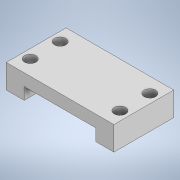
# Autodesk Inventor part: Controller_Strap
Saved by Autodesk Inventor 2022.3 (Build 263350000, 350)
## iProperties
Created: 2023-06-22
Part Number: Controller_Strap
Material: Generic
Document SubType Name: Modeling
Designer: natalie.jimenez
Density: 1 g/cm^3
Appearance: Default
Author: natalie.jimenez
Autodesk Inventor part; units mm, degrees
ref_plane "YZ Plane" through (0, 0, 0) normal (1, 0, 0) x (0, 1, 0)
ref_plane "XZ Plane" through (0, 0, 0) normal (0, 1, 0) x (-1, 0, 0)
ref_plane "XY Plane" through (0, 0, 0) normal (0, 0, 1) x (1, 0, 0)
sketch "Sketch1" plane through (0, 0, 0) normal (0, 1, 0) x (-1, 0, 0)
  line L0 (-11.43, -6.35) -> (11.43, -6.35)
  line L1 (11.43, -6.35) -> (11.43, 6.35)
  line L2 (11.43, 6.35) -> (-11.43, 6.35)
  line L3 (-11.43, 6.35) -> (-11.43, -6.35)
  line L4 (-11.43, -6.35) -> (11.43, 6.35) construction
  line L5 (11.43, -6.35) -> (-11.43, 6.35) construction
  point P0 (0, 0)
  point P1 (0, 0)
  dimension "d19" = 22.86
  dimension "d20" = 12.7
  constraints: 12 end point, 2 parallel, 1 coincident, 1 horizontal, 1 midpoint, 1 perpendicular
  measures "d19" distance between parallel lines of L3 L1
  measures "d20" distance between parallel lines of L0 L2
sketch "Sketch2" plane through (0, 0, 0) normal (0, 1, 0) x (-1, 0, 0)
  line L0 (9.525, 3.1634) -> (9.525, -3.1866) construction
  line L1 (9.525, -3.1866) -> (-9.525, -3.1866) construction
  line L2 (-9.525, -3.1866) -> (-9.525, 3.1634) construction
  line L3 (-9.525, 3.1634) -> (9.525, 3.1634) construction
  line L4 (9.525, 6.3268) -> (9.525, 3.1634) construction
  line L5 (-9.525, 3.1634) -> (-9.525, 6.5546) construction
  line L6 (11.43, -6.35) -> (11.43, 6.35) projected
  line L7 (-11.43, -6.35) -> (11.43, -6.35) projected
  line L8 (-11.43, 6.35) -> (-11.43, -6.35) projected
  line L9 (11.43, 6.35) -> (-11.43, 6.35) projected
  line L10 (9.525, -3.1866) -> (9.525, -6.35) construction
  point P0 (0, 0)
  dimension "d18" = 6.35
  dimension "d22" = 19.05
  dimension "d23" = 1.905
  dimension "d24" = 3.1634
  constraints: 14 end point, 4 perpendicular, 3 point on line, 2 collinear, 1 vertical
  measures "d18" distance between parallel lines of L1 L3
  measures "d22" distance between parallel lines of L2 L0
  measures "d23" distance between parallel lines of L6 L0
  measures "d24" distance between parallel lines of L1 L7
extrude "Extrusion1" add sketch "Sketch1" along normal blind 5.08
hole "Hole1" at (-9.525, 0, 3.1634) at (-9.525, 0, -3.1866) at (9.525, 0, -3.1866) at (9.525, 0, 3.1634) direction (0, 1, 0) diameter 2.4384 depth 5.08 clearance for "Flat Head Machine Screw (82)" size "#2" standard "Ansi Unified Screw Threads"
sketch "Sketch3" plane through (0, 0, 0) normal (0, -1, 0) x (1, 0, 0)
  line L0 (11.43, -6.35) -> (-11.43, -6.35) projected
  line L1 (7.62, 6.35) -> (-7.62, 6.35)
  line L2 (-7.62, 6.35) -> (-7.62, -6.35)
  line L3 (-7.62, -6.35) -> (7.62, -6.35)
  line L4 (7.62, -6.35) -> (7.62, 6.35)
  line L5 (7.62, 6.35) -> (-7.62, -6.35) construction
  line L6 (-7.62, 6.35) -> (7.62, -6.35) construction
  point P0 (0, 0)
  point P1 (7.62, -6.35)
  dimension "d34" = 15.24
  constraints: 12 end point, 2 midpoint, 2 parallel, 1 horizontal, 1 perpendicular, 1 point on line
  measures "d34" distance between parallel lines of L4 L2
extrude "Extrusion2" cut sketch "Sketch3" against normal blind 2.54
body "Solid1"
